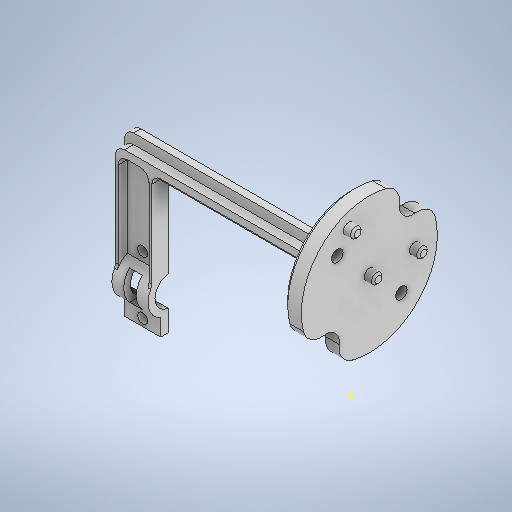
# Autodesk Inventor part: RobotarmHolder
Saved by Autodesk Inventor 2025.1 (Build 291241000, 241)
## iProperties
Created: 2025-03-06
Part Number: RobotarmHolder
Material: Generic
Document SubType Name: Modeling
Designer: frede
Density: 1 g/cm^3
Appearance: Default
Author: frede
Autodesk Inventor part; units mm, degrees
ref_plane "YZ Plane" through (0, 0, 0) normal (1, 0, 0) x (0, 1, 0)
ref_plane "XZ Plane" through (0, 0, 0) normal (0, 1, 0) x (-1, 0, 0)
ref_plane "XY Plane" through (0, 0, 0) normal (0, 0, 1) x (1, 0, 0)
sketch "Sketch1" plane through (0, 0, 0) normal (1, 0, 0) x (0, 1, 0)
  line L0 (20, 1) -> (20, 5)
  line L1 (-20, 5) -> (-20, 1)
  arc A0 (8.1892, 1) -> (-8.1892, 1) centre (0, 0) ccw
  line L2 (20, 5) -> (10.9087, 5)
  line L3 (-10.9087, 5) -> (-20, 5)
  line L4 (20, 1) -> (8.1892, 1)
  line L5 (-8.1892, 1) -> (-20, 1)
  arc A1 (10.9087, 5) -> (-10.9087, 5) centre (0, 0) ccw
  dimension "d2" = 40
  dimension "d5" = 8.25
  dimension "d6" = 40
  dimension "d7" = 12
  dimension "d8" = 20
  dimension "d9" = 1
  constraints: 12 end point, 4 point on circle, 2 centre point, 1 coincident, 1 parallel
  measures "d2" distance of L1.end L0.start
  measures "d5" radius of A0
  measures "d6" distance between parallel lines of L1 L0
  measures "d7" radius of A1
  measures "d8" distance from line of A0.centre L1
  measures "d9" distance from line of A0.centre L5
extrude "Extrusion1" add sketch "Sketch1" along normal blind 20
sketch "Sketch2" plane through (0, -20, 1) normal (0, 0, -1) x (-1, 0, 0)
  line L0 (0, 28.1892) -> (0, 40) projected
  line L1 (0, 40) -> (-20, 40) projected
  line L2 (-20, 28.1892) -> (-20, 40) projected
  line L3 (0, 28.1892) -> (-20, 28.1892) projected
  line L4 (0, 0) -> (0, 11.8108) projected
  line L5 (0, 11.8108) -> (-20, 11.8108) projected
  line L6 (-20, 0) -> (-20, 11.8108) projected
  line L7 (0, 0) -> (-20, 0) projected
  line L8 (-20, 11.8108) -> (-20, 28.1892) projected
  line L9 (0, 11.8108) -> (0, 28.1892) projected
  line L10 (-20, 28.1892) -> (0, 11.8108)
  line L11 (-20, 11.8108) -> (0, 28.1892)
  line L12 (-6.5, 28.1892) -> (-13.5, 28.1892)
  line L13 (-13.5, 28.1892) -> (-13.5, 11.8108)
  line L14 (-13.5, 11.8108) -> (-6.5, 11.8108)
  line L15 (-6.5, 11.8108) -> (-6.5, 28.1892)
  line L16 (-6.5, 28.1892) -> (-13.5, 11.8108) construction
  line L17 (-13.5, 28.1892) -> (-6.5, 11.8108) construction
  circle A0 centre (-10, 36) radius 2.75
  circle A1 centre (-10, 4) radius 2.75
  line L18 (-10, 36) -> (-10, 4)
  point P0 (0, 20)
  point P1 (-10, 20)
  dimension "d12" = 7
  dimension "d16" = 40
  dimension "d19" = 5.5
  dimension "d20" = 5.5
  dimension "d21" = 32
  dimension "d22" = 4
  dimension "d24" = 20
  dimension "d25" = 10
  constraints: 18 end point, 3 midpoint, 2 centre point, 2 parallel, 1 horizontal, 1 perpendicular, 1 point on line, 1 vertical
  measures "d12" distance of L14.end L13.end
  measures "d16" distance between parallel lines of L7 L1
  measures "d19" diameter of A0
  measures "d20" diameter of A1
  measures "d21" distance of L18.start L18.end
  measures "d22" distance from line of L1 L18.start
  measures "d24" distance between parallel lines of L0 L2
  measures "d25" distance between parallel lines of L2 L18
extrude "Extrusion2" cut sketch "Sketch2" against normal up to surface (11 mm away) contours L15 L11 L18 L3 | L15 L10 L11 | L18 L10 L13 L3 | L5 L18 L10 L15 | L11 L13 L10 | L18 L5 L13 L11 | A0 | A1
sketch "Sketch3" plane through (0, 20, 5) normal (0, 1, 0) x (1, 0, 0)
  line L0 (0, 4) -> (0, 0) projected
  line L1 (0, 0) -> (20, 0) projected
  line L2 (20, 4) -> (20, 0) projected
  line L3 (0, 4) -> (20, 4) projected
  point P0 (0, 5)
extrude "Extrusion3" add sketch "Sketch3" along normal blind 50
sketch "Sketch5" plane through (20, 0, 0) normal (1, 0, 0) x (0, 0, -1)
  line L0 (-5, 70) -> (-1, 70) projected
  line L1 (-1, 8.1892) -> (-1, 70) projected
  line L2 (-5, 70) -> (-1, 70)
  line L3 (-1, 70) -> (-1, 55)
  line L4 (-1, 55) -> (-5, 55)
  line L5 (-5, 55) -> (-5, 70)
  point P0 (0, 0)
  dimension "d28" = 15
  constraints: 8 end point, 2 parallel, 1 horizontal, 1 perpendicular, 1 point on line
  measures "d28" distance of L2.end L3.end
extrude "Extrusion4" add sketch "Sketch5" along normal blind 100
sketch "Sketch6" plane through (0, 10.9087, 5) normal (0, 0, 1) x (1, 0, 0)
  line L0 (120, 59.0913) -> (120, 44.0913) projected
  line L1 (0, 0) -> (0, 59.0913) projected
  line L2 (120, 53.5913) -> (0, 53.5913)
  line L3 (0, 53.5913) -> (0, 49.5913)
  line L4 (0, 49.5913) -> (120, 49.5913)
  line L5 (120, 49.5913) -> (120, 53.5913)
  line L6 (0, 59.0913) -> (120, 59.0913) projected
  line L7 (20, 44.0913) -> (120, 44.0913) projected
  line L8 (0, -2.7195) -> (6.5, -2.7195) projected
  line L9 (0, 49.5913) -> (1.5, 49.5913)
  line L10 (1.5, 49.5913) -> (1.5, -2.7195)
  line L11 (1.5, -2.7195) -> (0, -2.7195)
  line L12 (0, -2.7195) -> (0, 49.5913)
  line L13 (13.5, -2.7195) -> (20, -2.7195) projected
  line L14 (20, 49.5913) -> (18.5, 49.5913)
  line L15 (18.5, 49.5913) -> (18.5, -2.7195)
  line L16 (18.5, -2.7195) -> (20, -2.7195)
  line L17 (20, -2.7195) -> (20, 49.5913)
  point P0 (0, -10.9087)
  point P1 (0, 53.5913)
  point P2 (1.5, 49.5913)
  dimension "d31" = 4
  dimension "d32" = 15
  dimension "d33" = 5.5
  dimension "d36" = 1.5
  dimension "d37" = 1.5
  constraints: 24 end point, 6 parallel, 5 point on line, 3 horizontal, 3 perpendicular
  measures "d31" distance of L3.end L2.end
  measures "d32" distance between parallel lines of L6 L7
  measures "d33" distance between parallel lines of L6 L2
  measures "d36" distance of L10.end L11.end
  measures "d37" distance of L16.end L15.end
extrude "Extrusion5" add sketch "Sketch6" along normal blind 5 contours L0 L4 L1 L2 | L17 L13 L15 L4 | L4 L10 L8 L12 L1
sketch "Sketch7" plane through (0, 8.1892, 8.7714) normal (0, -1, 0) x (1, 0, 0)
  line L0 (1.5, 0) -> (0, 0) projected
  line L1 (1.5, 0) -> (1.5, 1.2286) projected
  line L2 (0, 1.2286) -> (1.5, 1.2286) projected
  line L3 (0, 0) -> (0, 1.2286) projected
  line L4 (20, 0) -> (18.5, 0) projected
  line L5 (20, 0) -> (20, 1.2286) projected
  line L6 (18.5, 1.2286) -> (20, 1.2286) projected
  line L7 (18.5, 0) -> (18.5, 1.2286) projected
  point P0 (0, -8.7714)
extrude "Extrusion6" add sketch "Sketch7" along normal up to surface round surface about axis through (0, 0, 0) along (1, 0, 0) radius 12 far side no
fillet "Fillet1" radius 5 7 edges at (0.75, 6.6332, 10) (19.25, 6.6332, 10) (1.5, 60.5, 7.5) (18.5, 60.5, 7.5) (20, 60.5, 7.5) (0, 64.5, 7.5) (0, 70, 3)
sketch "Sketch8" plane through (120, 0, 0) normal (1, 0, 0) x (0, 0, -1)
  point P0 (0, 0)
sketch "Sketch9" plane through (120, 0, 0) normal (1, 0, 0) x (0, 0, -1)
  circle A0 centre (0, 62.5) radius 37.5
  point P0 (0, 0)
  dimension "d41" = 75
  constraints: 1 centre point
  measures "d41" diameter of A0
extrude "Extrusion7" add sketch "Sketch9" along normal blind 10
fillet "Fillet2" radius 10 3 edges at (120, 70, 3) (120, 62.5, 10) (120, 55, 3)
sketch "Sketch10" plane through (130, 62.5, 0) normal (1, 0, 0) x (0, 0, -1)
  circle A0 centre (0, 0) radius 2.9
  point P0 (0, -62.5)
  dimension "d45" = 5.8
  constraints: 1 centre point
  measures "d45" diameter of A0
extrude "Extrusion8" add sketch "Sketch10" along normal blind 5
chamfer "Chamfer1" distance 1 angle 45 1 edges at (135, 62.5, 2.9)
sketch "Sketch11" plane through (130, 62.5, 0) normal (1, 0, 0) x (0, 0, -1)
  circle A0 centre (0, 0) radius 1.9 projected
  circle A1 centre (0, 0) radius 25
  circle A2 centre (-17.6777, 17.6777) radius 3.2
  line L0 (0, 0) -> (-37.5, 0)
  circle A3 centre (0, 0) radius 37.5 projected
  line L1 (-17.6777, 17.6777) -> (0, 0)
  circle A4 centre (17.6777, -17.6777) radius 3.2
  circle A5 centre (0, 0) radius 34
  line L2 (24.0416, 24.0416) -> (-24.0416, -24.0416)
  circle A6 centre (-24.0416, -24.0416) radius 7.5
  circle A7 centre (24.0416, 24.0416) radius 7.5
  point P0 (0, -62.5)
  dimension "d51" = 50
  dimension "d56" = 6.4
  dimension "d58" = 45
  dimension "d61" = 360
  dimension "d66" = 68
  dimension "d67" = 45
  dimension "d68" = 15
  dimension "d69" = 15
  constraints: 6 end point, 5 centre point, 4 coincident, 2 horizontal, 2 point on circle, 1 horizontal alignment, 9 other
  measures "d56" diameter of A2
  measures "d58" angle of L0 L1
  measures "d66" diameter of A5
  measures "d67" angle of L2 L0
  measures "d68" diameter of A6
  measures "d69" diameter of A7
extrude "Extrusion9" cut sketch "Sketch11" against normal up to surface (10 mm away) contours L1 A1 A2 | A2 A1 L1 | A1 A2 | A7 A5 L2 | L2 A5 A7 | A4 A1 | A1 A4 | A6 A5 L2 | L2 A5 A6 | A5 A7 A3 | A5 A6 A3 | A7 A3 | A3 A6
chamfer "Chamfer2" distance 2.5 angle 45 2 edges at (120, 89.0165, 26.5165) (120, 35.9835, -26.5165)
fillet "Fillet3" radius 10 4 edges at (126.25, 83.6543, -30.9636) (126.25, 93.4636, -21.1543) (126.25, 41.3457, 30.9636) (126.25, 31.5364, 21.1543)
chamfer "Chamfer3" distance 2.5 angle 45 6 edges at (120, 90.8041, -16.603) (120, 81.2383, -18.7383) (120, 79.103, -28.3041) (120, 43.7617, 18.7383) (120, 45.897, 28.3041) (120, 34.1959, 16.603)
sketch "Sketch12" plane through (130, 0, 0) normal (1, 0, 0) x (0, 0, -1)
  circle A0 centre (0, 62.5) radius 2.9 projected
  circle A1 centre (-17.6777, 80.1777) radius 3.2 projected
  circle A2 centre (0, 62.5) radius 25
  circle A3 centre (17.6777, 44.8223) radius 3.2 projected
  line L0 (-17.6777, 80.1777) -> (17.6777, 44.8223)
  circle A4 centre (0, 62.5) radius 30
  circle A5 centre (-11.4805, 90.2164) radius 2.9
  line L1 (0, 62.5) -> (-11.4805, 90.2164)
  circle A6 centre (25, 62.5) radius 2.9
  point P0 (0, 0)
  dimension "d75" = 60
  dimension "d74" = 50
  dimension "d76" = 5.8
  dimension "d77" = 157.5
  dimension "d78" = 5.8
  constraints: 4 end point, 3 centre point, 2 coincident, 2 point on circle, 3 other
  measures "d74" diameter of A2
  measures "d76" diameter of A5
  measures "d77" angle of L0 L1
  measures "d78" diameter of A6
extrude "Extrusion10" add sketch "Sketch12" along normal blind 5 contours A6 A2 | A2 A6 | A5 L1 A4 | A4 A5 | A4 L1 A5 picked at (-11.1992, 91.3014)
chamfer "Chamfer4" distance 1 angle 45 2 edges at (135, 90.2164, 14.3805) (135, 62.5, -22.1)
equation "\"d22\" = -0.5 * d21 + 0.5 * d16"
equation "\"d25\" = 0.5 * d24"
equation "\"d33\" = -0.5 * d31 + 0.5 * d32"
equation "\"d68\" = d69"
body "Solid1"
